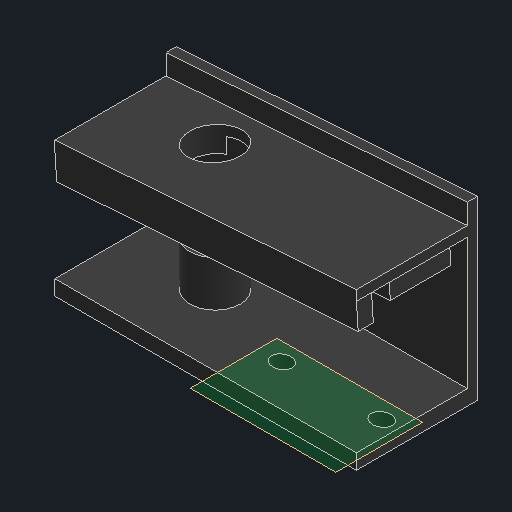
# Autodesk Inventor part: IMU_base
Saved by Autodesk Inventor 2026.1 (Build 301233020, 233B)
## iProperties
Created: 2025-12-04
Part Number: IMU_base
Material: 고무, 검은색
Document SubType Name: Modeling
Designer: jaewook
Density: 0.93 g/cm^3
Appearance: 고무 - 검은색
Author: jaewook
Autodesk Inventor part; units mm, degrees
ref_plane "YZ Plane" through (0, 0, 0) normal (1, 0, 0) x (0, 1, 0)
ref_plane "XZ Plane" through (0, 0, 0) normal (0, 1, 0) x (-1, 0, 0)
ref_plane "XY Plane" through (0, 0, 0) normal (0, 0, 1) x (1, 0, 0)
ref_plane "작업 평면1" through (-108.7402, -145.9081, -64.7043) normal (0, -1, 0) x (1, 0, 0)
sketch "스케치1" plane through (-108.7402, -145.9081, -64.7043) normal (0, -1, 0) x (1, 0, 0)
  ellipse E0 centre (-21.9712, -11.93) end of major axis (-19.8923, -11.93) minor radius 1.7957 projected
  ellipse E1 centre (-2.1698, -11.93) end of major axis (-0.091, -11.93) minor radius 1.7957 projected
  line L0 (-25.1804, -13.5798) -> (-25.1804, 0) projected
  ellipse E2 centre (0, 0) end of major axis (1.0394, 0) minor radius 0.8978 (1.0394, 0) -> (0, 0.8978) ccw projected
  line L1 (1.0394, 0) -> (1.0394, -13.5798) projected
  ellipse E3 centre (-0.2599, -13.5798) end of major axis (1.0394, -13.5798) minor radius 1.1223 (-0.2599, -14.7021) -> (1.0394, -13.5798) ccw projected
  line L2 (-0.2599, -14.7021) -> (-23.8811, -14.7021) projected
  ellipse E4 centre (-23.8811, -13.5798) end of major axis (-22.5818, -13.5798) minor radius 1.1223 (-25.1804, -13.5798) -> (-23.8811, -14.7021) ccw projected
  line L3 (-25.1804, -13.5798) -> (-25.1804, 0) projected
  ellipse E5 centre (-24.141, 0) end of major axis (-25.1804, 0) minor radius 0.8978 (-24.141, 0.8978) -> (-25.1804, 0) ccw projected
  line L4 (-24.141, 0.8978) -> (0, 0.8978) projected
  ellipse E6 centre (-21.9712, -11.93) end of major axis (-19.3726, -11.93) minor radius 2.2446 projected
  ellipse E7 centre (-2.1698, -11.93) end of major axis (0.4288, -11.93) minor radius 2.2446 projected
  ellipse E8 centre (-23.6213, -0.5275) end of major axis (-22.4194, -0.5275) minor radius 1.0381 projected
  ellipse E9 centre (-20.3211, -0.5275) end of major axis (-19.1192, -0.5275) minor radius 1.0381 projected
  ellipse E10 centre (-17.0208, -0.5275) end of major axis (-15.819, -0.5275) minor radius 1.0381 projected
  ellipse E11 centre (-13.7206, -0.5275) end of major axis (-12.5188, -0.5275) minor radius 1.0381 projected
  ellipse E12 centre (-10.4204, -0.5275) end of major axis (-9.2185, -0.5275) minor radius 1.0381 projected
  ellipse E13 centre (-7.1202, -0.5275) end of major axis (-5.9183, -0.5275) minor radius 1.0381 projected
  ellipse E14 centre (-3.8199, -0.5275) end of major axis (-2.6181, -0.5275) minor radius 1.0381 projected
  ellipse E15 centre (-0.5197, -0.5275) end of major axis (0.6821, -0.5275) minor radius 1.0381 projected
  line L5 (-25.1804, -3.7021) -> (1.0394, -3.7021)
  line L6 (1.0394, -27.7021) -> (-58.6804, -27.7021)
  line L7 (-58.6804, -27.7021) -> (-58.6804, -3.7021)
  line L8 (-58.6804, -3.7021) -> (1.0394, -3.7021)
  line L9 (1.0394, -3.7021) -> (1.0394, -27.7021)
  point P0 (108.7402, 64.7043)
  point P1 (-25.1804, -3.7021)
  point P2 (-25.1804, -3.7021)
  point P3 (1.0394, -13.5798)
  dimension "d0" = 11
  dimension "d3" = 33.5
  dimension "d4" = 13
  constraints: 10 end point, 2 collinear, 2 parallel, 2 perpendicular, 2 point on line, 1 horizontal, 4 other
  measures "d0" distance between parallel lines of L5 L2
  measures "d3" distance between parallel lines of L7 L0
  measures "d4" distance between parallel lines of L2 L6
extrude "돌출1" add sketch "스케치1" along normal blind 3 contours E4 L2 E3 L9 L6 L7 L8 L0 | L0 L5 L1 E3 L2 E4 | E6 | E7
sketch "스케치2" plane through (-108.7402, -145.9081, -64.7043) normal (0, 1, 0) x (1, 0, 0)
  line L0 (1.0394, 27.7021) -> (1.0394, 3.7021) projected
  line L1 (-58.6804, 27.7021) -> (1.0394, 27.7021) projected
  line L2 (-58.6804, 3.7021) -> (-58.6804, 27.7021) projected
  line L3 (1.0394, 27.7021) -> (-58.6804, 27.7021)
  line L4 (-58.6804, 27.7021) -> (-58.6804, 25.7021)
  line L5 (-58.6804, 25.7021) -> (1.0394, 25.7021)
  line L6 (1.0394, 25.7021) -> (1.0394, 27.7021)
  point P0 (108.7402, -64.7043)
  point P1 (1.0394, 25.7021)
  dimension "d5" = 2
  constraints: 8 end point, 2 parallel, 1 horizontal, 1 perpendicular, 1 point on line
  measures "d5" distance between parallel lines of L1 L5
extrude "돌출2" add sketch "스케치2" along normal blind 20
sketch "스케치4" plane through (-107.7008, -148.9081, -92.4064) normal (0, 0, -1) x (-1, 0, 0)
  line L0 (0, 23) -> (59.7199, 23) projected
  line L1 (0, 23) -> (0, 35)
  line L2 (0, 35) -> (42.7199, 35) construction
  line L3 (42.7199, 35) -> (42.7199, 32) construction
  line L4 (0, 35) -> (59.7199, 30.8062)
  line L5 (59.7199, 23) -> (59.7199, 40.663)
  point P0 (-107.7008, 148.9081)
  dimension "d11" = 42.7199
  dimension "d12" = 12
  dimension "d13" = 3
  constraints: 10 end point, 3 vertical, 2 point on line, 1 perpendicular
  measures "d11" distance of L1.end L2.end
  measures "d12" distance of L0.start L1.end
  measures "d13" distance of L2.end L3.end
extrude "돌출4" add sketch "스케치4" against normal blind 2
sketch "스케치5" plane through (-108.7402, -145.9081, -64.7043) normal (0, 1, 0) x (1, 0, 0)
  line L0 (1.0394, 3.7021) -> (-58.6804, 3.7021) projected
  line L1 (1.0394, 25.7021) -> (1.0394, 3.7021) projected
  circle A0 centre (-40.9606, 17.7021) radius 5
  point P0 (108.7402, -64.7043)
  dimension "d16" = 10
  dimension "d17" = 14
  dimension "d18" = 42
  constraints: 1 centre point
  measures "d16" diameter of A0
  measures "d17" distance from line of L0 A0.centre
  measures "d18" distance from line of L1 A0.centre
extrude "돌출5" add sketch "스케치5" along normal blind 9
sketch "스케치6" plane through (-167.4206, -145.9081, -90.4064) normal (0, 0, 1) x (1, 0, 0)
  line L0 (59.7199, 0) -> (59.7199, 32) projected
  line L1 (59.7199, 32) -> (0, 27.8062) projected
  line L2 (0, 0) -> (0, 27.8062) projected
  line L3 (59.7199, 25.9852) -> (0, 21.7914)
  line L4 (59.7199, 27.9901) -> (0, 23.7963)
  line L5 (0, 23.7963) -> (0, 21.7914)
  line L6 (59.7199, 27.9901) -> (59.7199, 25.9852)
  point P0 (167.4206, 145.9081)
  point P1 (0, 23.7963)
  dimension "d21" = 6
  dimension "d22" = 2
  constraints: 8 end point, 3 parallel, 2 point on line, 1 collinear
  measures "d21" distance between parallel lines of L3 L1
  measures "d22" distance between parallel lines of L3 L4
extrude "돌출6" add sketch "스케치6" along normal up to surface (22 mm away) contours L3 L2 L4 L0
sketch "스케치11" plane through (-167.4206, -124.1167, -90.4064) normal (0.0701, -0.9975, 0) x (0.9975, 0.0701, 0)
  line L0 (59.8669, 22) -> (0, 22) projected
  line L1 (0, 0) -> (0, 22) projected
  line L2 (59.8669, 0) -> (0, 0) projected
  line L3 (59.8669, 0) -> (59.8669, 22) projected
  line L4 (0, 15.5) -> (59.8669, 15.5)
  line L5 (57.8365, 22) -> (-1.7367, 22) projected
  line L6 (0, 3.5) -> (59.8669, 3.5)
  point P0 (175.704, 90.4064)
  dimension "d36" = 6.5
  dimension "d39" = 3.5
  constraints: 4 end point, 4 point on line, 2 parallel, 1 horizontal
  measures "d36" distance between parallel lines of L4 L0
  measures "d39" distance between parallel lines of L2 L6
extrude "돌출11" add sketch "스케치11" along normal blind 3 contours L3 L6 L1 L4
sketch "스케치7" plane through (-149.7008, -136.9081, -82.4064) normal (0, 1, 0) x (1, 0, 0)
  circle A0 centre (0, 0) radius 5 projected
  circle A1 centre (0, 0) radius 1.9
  point P0 (149.7008, -82.4064)
  dimension "d25" = 3.8
  constraints: 1 centre point, 1 coincident
  measures "d25" diameter of A1
extrude "돌출7" cut sketch "스케치7" against normal through all contours A1
sketch "스케치8" plane through (-149.7008, -136.9081, -82.4064) normal (0, 1, 0) x (1, 0, 0)
  circle A0 centre (0, 0) radius 5 projected
  point P0 (149.7008, -82.4064)
extrude "돌출8" cut sketch "스케치8" along normal blind 16.75
sketch "스케치9" plane through (-167.4206, -124.1167, -90.4064) normal (0.0701, -0.9975, 0) x (0.9975, 0.0701, 0)
  line L0 (59.8669, 22) -> (0, 22) projected
  line L1 (0, 0) -> (0, 22) projected
  line L2 (59.8669, 0) -> (59.8669, 22) projected
  line L3 (0, 19) -> (59.8669, 19)
  point P0 (175.704, 90.4064)
  dimension "d30" = 3
  constraints: 2 end point, 2 point on line, 1 parallel
  measures "d30" distance between parallel lines of L3 L0
extrude "돌출9" add sketch "스케치9" along normal blind 5
